Autodesk Inventor part; units mm, degrees
(part 3 of 3)
sketch "Sketch57" plane through (0, 10, 0) normal (0, 1, 0) x (1, 0, 0)
  line L0 (-74.5, 125.8) -> (-66.5, 125.8) projected
  line L1 (-83.25, 131.7) -> (2.25, 131.7) projected
  line L2 (-74.5, 125.8) -> (-66.5, 125.8)
  line L3 (-66.5, 125.8) -> (-66.5, 131.7)
  line L4 (-66.5, 131.7) -> (-74.5, 131.7)
  line L5 (-74.5, 131.7) -> (-74.5, 125.8)
  line L6 (-66.5, 9.8) -> (-74.5, 9.8) projected
  line L7 (2.25, 3.9) -> (-83.25, 3.9) projected
  line L8 (-74.5, 9.8) -> (-66.5, 9.8)
  line L9 (-66.5, 9.8) -> (-66.5, 3.9)
  line L10 (-66.5, 3.9) -> (-74.5, 3.9)
  line L11 (-74.5, 3.9) -> (-74.5, 9.8)
  line L12 (-44.5, 125.8) -> (-36.5, 125.8) projected
  line L13 (-44.5, 125.8) -> (-36.5, 125.8)
  line L14 (-36.5, 125.8) -> (-36.5, 131.7)
  line L15 (-36.5, 131.7) -> (-44.5, 131.7)
  line L16 (-44.5, 131.7) -> (-44.5, 125.8)
  line L17 (-14.5, 125.8) -> (-6.5, 125.8) projected
  line L18 (-14.5, 125.8) -> (-6.5, 125.8)
  line L19 (-6.5, 125.8) -> (-6.5, 131.7)
  line L20 (-6.5, 131.7) -> (-14.5, 131.7)
  line L21 (-14.5, 131.7) -> (-14.5, 125.8)
  line L22 (-44.5, 9.8) -> (-44.5, 125.8) projected
  line L23 (-44.5, 9.8) -> (-36.5, 9.8)
  line L24 (-36.5, 9.8) -> (-36.5, 3.9)
  line L25 (-36.5, 3.9) -> (-44.5, 3.9)
  line L26 (-44.5, 3.9) -> (-44.5, 9.8)
  line L27 (-6.5, 9.8) -> (-14.5, 9.8) projected
  line L28 (-14.5, 9.8) -> (-6.5, 9.8)
  line L29 (-6.5, 9.8) -> (-6.5, 3.9)
  line L30 (-6.5, 3.9) -> (-14.5, 3.9)
  line L31 (-14.5, 3.9) -> (-14.5, 9.8)
  point P0 (0, 0)
  dimension "d516" = 8
  dimension "d517" = 8
  constraints: 48 end point, 12 parallel, 9 point on line, 6 horizontal, 6 perpendicular
  measures "d516" distance of L4.end L3.end
  measures "d517" distance of L15.end L14.end
extrude "Extrusion53" add sketch "Sketch57" against normal blind 5
sketch "Sketch59" plane through (0, 10, 0) normal (0, 1, 0) x (1, 0, 0)
  point P0 (0, 0)
sketch "Sketch60" plane through (0, 10, 0) normal (0, 1, 0) x (1, 0, 0)
  line L0 (-66.5, 131.7) -> (-66.5, 3.9) projected
  line L1 (-66.5, 131.7) -> (-74.5, 131.7) projected
  line L2 (-74.5, 3.9) -> (-74.5, 131.7) projected
  line L3 (-74.5, 3.9) -> (-66.5, 3.9) projected
  line L4 (-36.5, 131.7) -> (-36.5, 3.9) projected
  line L5 (-36.5, 131.7) -> (-44.5, 131.7) projected
  line L6 (-44.5, 3.9) -> (-44.5, 131.7) projected
  line L7 (-44.5, 3.9) -> (-36.5, 3.9) projected
  line L8 (-6.5, 131.7) -> (-6.5, 3.9) projected
  line L9 (-6.5, 131.7) -> (-14.5, 131.7) projected
  line L10 (-14.5, 3.9) -> (-14.5, 131.7) projected
  line L11 (-14.5, 3.9) -> (-6.5, 3.9) projected
  point P0 (0, 0)
extrude "Extrusion54" add sketch "Sketch60" along normal blind 3
sketch "Sketch62" plane through (0, 13, 0) normal (0, 1, 0) x (1, 0, 0)
  line L0 (-66.5, 131.7) -> (-66.5, 3.9) projected
  line L1 (-74.5, 3.9) -> (-74.5, 131.7) projected
  line L2 (-66.5, 131.7) -> (-74.5, 131.7)
  line L3 (-74.5, 131.7) -> (-74.5, 108.7)
  line L4 (-74.5, 108.7) -> (-66.5, 108.7)
  line L5 (-66.5, 108.7) -> (-66.5, 131.7)
  line L6 (-74.5, 108.7) -> (-66.5, 108.7)
  line L7 (-66.5, 108.7) -> (-66.5, 85.7)
  line L8 (-66.5, 85.7) -> (-74.5, 85.7)
  line L9 (-74.5, 85.7) -> (-74.5, 108.7)
  line L10 (-74.5, 85.7) -> (-66.5, 85.7)
  line L11 (-66.5, 85.7) -> (-66.5, 62.7)
  line L12 (-66.5, 62.7) -> (-74.5, 62.7)
  line L13 (-74.5, 62.7) -> (-74.5, 85.7)
  line L14 (-74.5, 62.7) -> (-66.5, 62.7)
  line L15 (-66.5, 62.7) -> (-66.5, 39.7)
  line L16 (-66.5, 39.7) -> (-74.5, 39.7)
  line L17 (-74.5, 39.7) -> (-74.5, 62.7)
  line L18 (-66.5, 39.7) -> (-74.5, 39.7)
  line L19 (-74.5, 39.7) -> (-74.5, 16.7)
  line L20 (-74.5, 16.7) -> (-66.5, 16.7)
  line L21 (-66.5, 16.7) -> (-66.5, 39.7)
  line L22 (-83.25, 131.7) -> (2.25, 131.7) projected
  line L23 (-83.25, 131.7) -> (-76.85, 131.7)
  line L24 (-76.85, 131.7) -> (-76.85, 125.3)
  line L25 (-76.85, 125.3) -> (-83.25, 125.3)
  line L26 (-83.25, 125.3) -> (-83.25, 131.7)
  line L27 (2.25, 131.7) -> (2.25, 3.9) projected
  line L28 (2.25, 3.9) -> (-4.15, 3.9)
  line L29 (-4.15, 3.9) -> (-4.15, 10.3)
  line L30 (-4.15, 10.3) -> (2.25, 10.3)
  line L31 (2.25, 10.3) -> (2.25, 3.9)
  line L32 (2.25, 3.9) -> (-83.25, 3.9)
  line L33 (-83.25, 3.9) -> (-83.25, 131.7)
  line L34 (-83.25, 131.7) -> (2.25, 131.7)
  line L35 (2.25, 131.7) -> (2.25, 3.9)
  line L36 (-4.15, 10.3) -> (-76.85, 10.3)
  line L37 (-76.85, 10.3) -> (-76.85, 125.3)
  line L38 (-76.85, 125.3) -> (-4.15, 125.3)
  line L39 (-4.15, 125.3) -> (-4.15, 10.3)
  point P0 (0, 0)
  dimension "d558" = 23
  dimension "d559" = 23
  dimension "d560" = 23
  dimension "d561" = 23
  dimension "d562" = 23
  dimension "d563" = 6.4
  dimension "d564" = 6.4
  dimension "d565" = 6.4
  dimension "d566" = 6.4
  constraints: 72 end point, 18 parallel, 9 horizontal, 9 perpendicular, 5 point on line
  measures "d558" distance of L3.end L2.end
  measures "d559" distance of L6.end L7.end
  measures "d560" distance of L10.end L11.end
  measures "d561" distance of L14.end L15.end
  measures "d562" distance of L19.end L18.end
  measures "d563" distance of L24.end L25.end
  measures "d564" distance of L23.end L24.end
  measures "d565" distance of L29.end L30.end
  measures "d566" distance of L28.end L29.end
extrude "Extrusion55" cut sketch "Sketch62" against normal blind 8 contours L38 L1 L2 L0 | L0 L22 L27 L30 L39 L38 | L38 L24 L22 L1 | L25 L26 L22 L24 | L37 L36 L1 L32 L33 L25 | L30 L27 L28 L29 | L29 L32 L0 L36 | L0 L32 L1 L36
sketch "Sketch63" plane through (0, 13, 0) normal (0, 1, 0) x (1, 0, 0)
  line L0 (-66.5, 125.3) -> (-74.5, 125.3) projected
  line L1 (-6.5, 125.3) -> (-6.5, 10.3) projected
  line L2 (-74.5, 125.3) -> (-6.5, 125.3)
  line L3 (-6.5, 125.3) -> (-6.5, 102.3)
  line L4 (-6.5, 102.3) -> (-74.5, 102.3)
  line L5 (-74.5, 102.3) -> (-74.5, 125.3)
  line L6 (-74.5, 125.3) -> (-74.5, 10.3) projected
  line L7 (-6.5, 102.3) -> (-74.5, 102.3)
  line L8 (-74.5, 102.3) -> (-74.5, 79.3)
  line L9 (-74.5, 79.3) -> (-6.5, 79.3)
  line L10 (-6.5, 79.3) -> (-6.5, 102.3)
  line L11 (-74.5, 79.3) -> (-6.5, 79.3)
  line L12 (-6.5, 79.3) -> (-6.5, 56.3)
  line L13 (-6.5, 56.3) -> (-74.5, 56.3)
  line L14 (-74.5, 56.3) -> (-74.5, 79.3)
  line L15 (-6.5, 56.3) -> (-74.5, 56.3)
  line L16 (-74.5, 56.3) -> (-74.5, 33.3)
  line L17 (-74.5, 33.3) -> (-6.5, 33.3)
  line L18 (-6.5, 33.3) -> (-6.5, 56.3)
  line L19 (-74.5, 33.3) -> (-6.5, 33.3)
  line L20 (-6.5, 33.3) -> (-6.5, 10.3)
  line L21 (-6.5, 10.3) -> (-74.5, 10.3)
  line L22 (-74.5, 10.3) -> (-74.5, 33.3)
  line L23 (-66.5, 10.3) -> (-66.5, 125.3) projected
  line L24 (-74.5, 125.3) -> (-66.5, 125.3)
  line L25 (-66.5, 125.3) -> (-66.5, 102.3)
  line L26 (-66.5, 102.3) -> (-74.5, 102.3)
  line L27 (-74.5, 102.3) -> (-74.5, 125.3)
  line L28 (-74.5, 102.3) -> (-66.5, 102.3)
  line L29 (-66.5, 102.3) -> (-66.5, 79.3)
  line L30 (-66.5, 79.3) -> (-74.5, 79.3)
  line L31 (-74.5, 79.3) -> (-74.5, 102.3)
  line L32 (-74.5, 79.3) -> (-66.5, 79.3)
  line L33 (-66.5, 79.3) -> (-66.5, 56.3)
  line L34 (-66.5, 56.3) -> (-74.5, 56.3)
  line L35 (-74.5, 56.3) -> (-74.5, 79.3)
  line L36 (-74.5, 56.3) -> (-66.5, 56.3)
  line L37 (-66.5, 56.3) -> (-66.5, 33.3)
  line L38 (-66.5, 33.3) -> (-74.5, 33.3)
  line L39 (-74.5, 33.3) -> (-74.5, 56.3)
  line L40 (-74.5, 33.3) -> (-66.5, 33.3)
  line L41 (-66.5, 33.3) -> (-66.5, 10.3)
  line L42 (-66.5, 10.3) -> (-74.5, 10.3)
  line L43 (-74.5, 10.3) -> (-74.5, 33.3)
  line L44 (-44.5, 125.3) -> (-44.5, 10.3) projected
  line L45 (-36.5, 125.3) -> (-36.5, 10.3) projected
  line L46 (-44.5, 10.3) -> (-36.5, 10.3)
  line L47 (-36.5, 10.3) -> (-36.5, 33.3)
  line L48 (-36.5, 33.3) -> (-44.5, 33.3)
  line L49 (-44.5, 33.3) -> (-44.5, 10.3)
  line L50 (-44.5, 56.3) -> (-36.5, 56.3)
  line L51 (-36.5, 56.3) -> (-36.5, 33.3)
  line L52 (-36.5, 33.3) -> (-44.5, 33.3)
  line L53 (-44.5, 33.3) -> (-44.5, 56.3)
  line L54 (-44.5, 56.3) -> (-36.5, 56.3)
  line L55 (-36.5, 56.3) -> (-36.5, 79.3)
  line L56 (-36.5, 79.3) -> (-44.5, 79.3)
  line L57 (-44.5, 79.3) -> (-44.5, 56.3)
  line L58 (-44.5, 79.3) -> (-36.5, 79.3)
  line L59 (-36.5, 79.3) -> (-36.5, 102.3)
  line L60 (-36.5, 102.3) -> (-44.5, 102.3)
  line L61 (-44.5, 102.3) -> (-44.5, 79.3)
  line L62 (-44.5, 102.3) -> (-36.5, 102.3)
  line L63 (-36.5, 102.3) -> (-36.5, 125.3)
  line L64 (-36.5, 125.3) -> (-44.5, 125.3)
  line L65 (-44.5, 125.3) -> (-44.5, 102.3)
  line L66 (-14.5, 125.3) -> (-14.5, 10.3) projected
  line L67 (-6.5, 125.3) -> (-14.5, 125.3)
  line L68 (-14.5, 125.3) -> (-14.5, 102.3)
  line L69 (-14.5, 102.3) -> (-6.5, 102.3)
  line L70 (-6.5, 102.3) -> (-6.5, 125.3)
  line L71 (-6.5, 79.3) -> (-14.5, 79.3)
  line L72 (-14.5, 79.3) -> (-14.5, 102.3)
  line L73 (-14.5, 102.3) -> (-6.5, 102.3)
  line L74 (-6.5, 102.3) -> (-6.5, 79.3)
  line L75 (-14.5, 79.3) -> (-6.5, 79.3)
  line L76 (-6.5, 79.3) -> (-6.5, 56.3)
  line L77 (-6.5, 56.3) -> (-14.5, 56.3)
  line L78 (-14.5, 56.3) -> (-14.5, 79.3)
  line L79 (-14.5, 56.3) -> (-6.5, 56.3)
  line L80 (-6.5, 56.3) -> (-6.5, 33.3)
  line L81 (-6.5, 33.3) -> (-14.5, 33.3)
  line L82 (-14.5, 33.3) -> (-14.5, 56.3)
  line L83 (-14.5, 33.3) -> (-6.5, 33.3)
  line L84 (-6.5, 33.3) -> (-6.5, 10.3)
  line L85 (-6.5, 10.3) -> (-14.5, 10.3)
  line L86 (-14.5, 10.3) -> (-14.5, 33.3)
  line L87 (-70.5, 125.3) -> (-74.5, 121.3)
  line L88 (-70.5, 125.3) -> (-64.8431, 125.3) construction
  line L89 (-74.5, 121.3) -> (-70.5, 125.3)
  line L90 (-70.5, 125.3) -> (-66.5, 121.3)
  line L91 (-70.5, 102.3) -> (-66.5, 106.3)
  line L92 (-70.5, 102.3) -> (-74.5, 106.3)
  line L93 (-70.5, 102.3) -> (-66.5, 98.3)
  line L94 (-70.5, 102.3) -> (-74.5, 98.3)
  line L95 (-70.5, 79.3) -> (-66.5, 83.3)
  line L96 (-70.5, 79.3) -> (-74.5, 83.3)
  line L97 (-70.5, 79.3) -> (-66.5, 75.3)
  line L98 (-70.5, 79.3) -> (-74.5, 75.3)
  line L99 (-70.5, 56.3) -> (-66.5, 60.3)
  line L100 (-70.5, 56.3) -> (-74.5, 60.3)
  line L101 (-70.5, 56.3) -> (-74.5, 52.3)
  line L102 (-70.5, 56.3) -> (-66.5, 52.3)
  line L103 (-70.5, 33.3) -> (-66.5, 37.3)
  line L104 (-70.5, 33.3) -> (-74.5, 37.3)
  line L105 (-70.5, 33.3) -> (-74.5, 29.3)
  line L106 (-70.5, 33.3) -> (-66.5, 29.3)
  line L107 (-70.5, 10.3) -> (-74.5, 14.3)
  line L108 (-70.5, 10.3) -> (-66.5, 14.3)
  line L109 (-36.5, 125.3) -> (-44.5, 125.3) projected
  line L110 (-40.5, 125.3) -> (-44.5, 121.3)
  line L111 (-40.5, 125.3) -> (-36.5, 121.3)
  line L112 (-40.5, 102.3) -> (-36.5, 106.3)
  line L113 (-40.5, 102.3) -> (-44.5, 106.3)
  line L114 (-40.5, 102.3) -> (-44.5, 98.3)
  line L115 (-40.5, 102.3) -> (-36.5, 98.3)
  line L116 (-40.5, 79.3) -> (-44.5, 83.3)
  line L117 (-40.5, 79.3) -> (-36.5, 83.3)
  line L118 (-36.5, 83.3) -> (-40.5, 79.3)
  line L119 (-44.5, 75.3) -> (-40.5, 79.3)
  line L120 (-36.5, 75.3) -> (-40.5, 79.3)
  line L121 (-40.5, 56.3) -> (-36.5, 60.3)
  line L122 (-40.5, 56.3) -> (-44.5, 60.3)
  line L123 (-40.5, 56.3) -> (-44.5, 52.3)
  line L124 (-40.5, 56.3) -> (-36.5, 52.3)
  line L125 (-40.5, 33.3) -> (-36.5, 37.3)
  line L126 (-40.5, 33.3) -> (-44.5, 37.3)
  line L127 (-40.5, 33.3) -> (-44.5, 29.3)
  line L128 (-40.5, 33.3) -> (-36.5, 29.3)
  line L129 (-40.5, 10.3) -> (-36.5, 14.3)
  line L130 (-40.5, 10.3) -> (-44.5, 14.3)
  line L131 (-6.5, 125.3) -> (-14.5, 125.3) projected
  line L132 (-10.5, 125.3) -> (-14.5, 121.3)
  line L133 (-10.5, 125.3) -> (-6.5, 121.3)
  line L134 (-10.5, 102.3) -> (-6.5, 106.3)
  line L135 (-10.5, 102.3) -> (-4.8431, 102.3) construction
  line L136 (-6.5, 106.3) -> (-10.5, 102.3)
  line L137 (-14.5, 106.3) -> (-10.5, 102.3)
  line L138 (-10.5, 102.3) -> (-14.5, 98.3)
  line L139 (-10.5, 102.3) -> (-6.5, 98.3)
  line L140 (-10.5, 79.3) -> (-6.5, 83.3)
  line L141 (-10.5, 79.3) -> (-14.5, 83.3)
  line L142 (-10.5, 79.3) -> (-14.5, 75.3)
  line L143 (-10.5, 79.3) -> (-6.5, 75.3)
  line L144 (-10.5, 56.3) -> (-6.5, 60.3)
  line L145 (-10.5, 56.3) -> (-4.8431, 56.3) construction
  line L146 (-6.5, 60.3) -> (-10.5, 56.3)
  line L147 (-14.5, 60.3) -> (-10.5, 56.3)
  line L148 (-10.5, 56.3) -> (-14.5, 52.3)
  line L149 (-10.5, 56.3) -> (-6.5, 52.3)
  line L150 (-10.5, 33.3) -> (-6.5, 37.3)
  line L151 (-10.5, 33.3) -> (-14.5, 37.3)
  line L152 (-10.5, 33.3) -> (-14.5, 29.3)
  line L153 (-10.5, 33.3) -> (-6.5, 29.3)
  line L154 (-14.5, 10.3) -> (-6.5, 10.3) projected
  line L155 (-10.5, 10.3) -> (-6.5, 14.3)
  line L156 (-10.5, 10.3) -> (-14.5, 14.3)
  point P0 (0, 0)
  dimension "d569" = 23
  dimension "d570" = 23
  dimension "d571" = 23
  dimension "d572" = 23
  dimension "d573" = 23
  dimension "d574" = 135
  dimension "d575" = 45
  dimension "d576" = 45
  constraints: 294 end point, 109 point on line, 53 equal length, 48 perpendicular, 23 horizontal, 18 midpoint
  measures "d569" distance of L2.end L3.end
  measures "d570" distance of L8.end L7.end
  measures "d571" distance of L11.end L12.end
  measures "d572" distance of L16.end L15.end
  measures "d573" distance of L19.end L20.end
  measures "d574" angle of L87 L88
  measures "d575" angle of L135 L134
  measures "d576" angle of L145 L144
extrude "Extrusion56" cut sketch "Sketch63" against normal blind 3 contours L90 L23 L91 L92 L5 L87 | L111 L45 L112 L113 L44 L110 | L93 L23 L95 L96 L6 L94 | L115 L45 L117 L116 L44 L114 | L133 L1 L134 L137 L66 L132 | L97 L23 L99 L100 L6 L98 | L139 L1 L140 L141 L66 L138 | L120 L45 L121 L122 L44 L119 | L143 L1 L144 L147 L66 L142 | L102 L23 L103 L104 L6 L101 | L124 L45 L125 L126 L44 L123 | L149 L1 L150 L151 L66 L148 | L106 L23 L108 L107 L6 L105 | L128 L45 L129 L130 L44 L127 | L153 L1 L155 L156 L66 L152
sketch "Sketch64" plane through (0, 13, 0) normal (0, 1, 0) x (1, 0, 0)
  line L0 (-83.25, 131.7) -> (2.25, 131.7) projected
  line L1 (2.25, 131.7) -> (2.25, 3.9) projected
  line L2 (-83.25, 131.7) -> (2.25, 131.7)
  line L3 (2.25, 131.7) -> (2.25, 3.9)
  line L4 (2.25, 3.9) -> (-83.25, 3.9)
  line L5 (-83.25, 3.9) -> (-83.25, 131.7)
  point P0 (0, 0)
  constraints: 8 end point, 2 parallel, 1 horizontal, 1 perpendicular
extrude "Extrusion57" cut sketch "Sketch64" against normal blind 10
sketch "Sketch65" plane through (0, 3, 0) normal (0, 1, 0) x (1, 0, 0)
  line L0 (2.25, 3.9) -> (-83.25, 3.9) projected
  line L1 (2.25, 131.7) -> (2.25, 3.9) projected
  line L2 (-83.25, 131.7) -> (2.25, 131.7) projected
  line L3 (-83.25, 3.9) -> (-83.25, 131.7) projected
  point P0 (0, 0)
extrude "Extrusion58" add sketch "Sketch65" along normal blind 5
sketch "Sketch66" plane through (0, 8, 0) normal (0, 1, 0) x (1, 0, 0)
  point P0 (0, 0)
sketch "Sketch67" plane through (0, 8, 0) normal (0, 1, 0) x (1, 0, 0)
  point P0 (0, 0)
sketch "Sketch68" plane through (0, 8, 0) normal (0, 1, 0) x (1, 0, 0)
  line L0 (-83.25, 3.9) -> (-83.25, 131.7) projected
  line L1 (-83.25, 131.7) -> (2.25, 131.7) projected
  line L2 (-83.25, 3.9) -> (2.25, 3.9)
  line L3 (2.25, 3.9) -> (2.25, 131.7)
  line L4 (2.25, 131.7) -> (-83.25, 131.7)
  line L5 (-83.25, 131.7) -> (-83.25, 3.9)
  line L6 (2.25, 3.9) -> (-83.25, 3.9) projected
  line L7 (-40.5, 3.9) -> (-83.25, 3.9)
  line L8 (-83.25, 3.9) -> (-83.25, 131.7)
  line L9 (-83.25, 131.7) -> (-40.5, 131.7)
  line L10 (-40.5, 131.7) -> (-40.5, 3.9)
  line L11 (-83.25, 3.9) -> (-61.875, 3.9)
  line L12 (-61.875, 3.9) -> (-61.875, 131.7)
  line L13 (-61.875, 131.7) -> (-83.25, 131.7)
  line L14 (-83.25, 131.7) -> (-83.25, 3.9)
  line L15 (-61.875, 3.9) -> (-63.145, 3.9)
  line L16 (-63.145, 3.9) -> (-63.145, 131.7)
  line L17 (-63.145, 131.7) -> (-61.875, 131.7)
  line L18 (-61.875, 131.7) -> (-61.875, 3.9)
  line L19 (-63.145, 131.7) -> (-60.605, 131.7)
  line L20 (-60.605, 131.7) -> (-60.605, 3.9)
  line L21 (-60.605, 3.9) -> (-63.145, 3.9)
  line L22 (-63.145, 3.9) -> (-63.145, 131.7)
  line L23 (-63.145, 67.8) -> (-60.605, 67.8)
  line L24 (-60.605, 67.8) -> (-60.605, 86.85)
  line L25 (-60.605, 86.85) -> (-63.145, 86.85)
  line L26 (-63.145, 86.85) -> (-63.145, 67.8)
  line L27 (-60.605, 86.85) -> (-63.145, 86.85)
  line L28 (-63.145, 86.85) -> (-63.145, 48.75)
  line L29 (-63.145, 48.75) -> (-60.605, 48.75)
  line L30 (-60.605, 48.75) -> (-60.605, 86.85)
  point P0 (0, 0)
  dimension "d583" = 1.27
  dimension "d584" = 2.54
  dimension "d585" = 19.05
  dimension "d586" = 2.54
  dimension "d587" = 38.1
  constraints: 56 end point, 14 parallel, 7 horizontal, 7 perpendicular, 3 midpoint, 3 point on line
  measures "d583" distance of L16.end L17.end
  measures "d584" distance of L20.end L21.end
  measures "d585" distance of L24.end L23.end
  measures "d586" distance of L29.end L28.end
  measures "d587" distance of L28.end L27.end
extrude "Extrusion59" add sketch "Sketch68" along normal blind 50.8 contours L16 L23 L12 L29 | L25 L12 L23 L16 | L12 L23 L20 L29 | L25 L20 L23 L12
sketch "Sketch69" plane through (-63.145, 8, -86.85) normal (-1, 0, 0) x (0, 0, 1)
  line L0 (0, 50.8) -> (4.9276, 50.8)
  line L1 (4.9276, 50.8) -> (4.9276, 45.8724)
  line L2 (4.9276, 45.8724) -> (0, 45.8724)
  line L3 (0, 45.8724) -> (0, 50.8)
  line L4 (0, 50.8) -> (38.1, 50.8) projected
  line L5 (38.1, 50.8) -> (0, 50.8)
  line L6 (0, 50.8) -> (0, 12.7)
  line L7 (0, 12.7) -> (38.1, 12.7)
  line L8 (38.1, 12.7) -> (38.1, 50.8)
  line L9 (0, 12.7) -> (4.9276, 12.7)
  line L10 (4.9276, 12.7) -> (4.9276, 17.6276)
  line L11 (4.9276, 17.6276) -> (0, 17.6276)
  line L12 (0, 17.6276) -> (0, 12.7)
  line L13 (38.1, 12.7) -> (33.1724, 12.7)
  line L14 (33.1724, 12.7) -> (33.1724, 17.6276)
  line L15 (33.1724, 17.6276) -> (38.1, 17.6276)
  line L16 (38.1, 17.6276) -> (38.1, 12.7)
  line L17 (38.1, 0) -> (38.1, 50.8) projected
  line L18 (38.1, 50.8) -> (33.1724, 50.8)
  line L19 (33.1724, 50.8) -> (33.1724, 45.8724)
  line L20 (33.1724, 45.8724) -> (38.1, 45.8724)
  line L21 (38.1, 45.8724) -> (38.1, 50.8)
  line L22 (38.1, 50.8) -> (19.05, 50.8)
  line L23 (19.05, 50.8) -> (19.05, 31.75)
  line L24 (19.05, 31.75) -> (38.1, 31.75)
  line L25 (38.1, 31.75) -> (38.1, 50.8)
  circle A0 centre (19.05, 31.75) radius 11.43
  circle A1 centre (33.1724, 45.8724) radius 1.27
  circle A2 centre (4.9276, 45.8724) radius 1.27
  circle A3 centre (4.9276, 17.6276) radius 1.27
  circle A4 centre (33.1724, 17.6276) radius 1.27
  point P0 (86.85, -8)
  dimension "d590" = 4.9276
  dimension "d591" = 4.9276
  dimension "d592" = 38.1
  dimension "d593" = 38.1
  dimension "d594" = 4.9276
  dimension "d595" = 4.9276
  dimension "d596" = 4.9276
  dimension "d597" = 4.9276
  dimension "d598" = 4.9276
  dimension "d599" = 4.9276
  dimension "d600" = 19.05
  dimension "d601" = 19.05
  dimension "d602" = 22.86
  dimension "d603" = 2.54
  dimension "d604" = 2.54
  dimension "d605" = 2.54
  dimension "d606" = 2.54
  constraints: 48 end point, 12 parallel, 6 horizontal, 6 perpendicular, 5 centre point, 5 coincident
  measures "d590" distance of L1.end L2.end
  measures "d591" distance of L0.end L1.end
  measures "d592" distance of L7.end L6.end
  measures "d593" distance of L6.end L5.end
  measures "d594" distance of L11.end L10.end
  measures "d595" distance of L10.end L9.end
  measures "d596" distance of L14.end L15.end
  measures "d597" distance of L13.end L14.end
  measures "d598" distance of L20.end L19.end
  measures "d599" distance of L19.end L18.end
  measures "d600" distance of L24.end L23.end
  measures "d601" distance of L23.end L22.end
  measures "d602" diameter of A0
  measures "d603" diameter of A1
  measures "d604" diameter of A2
  measures "d605" diameter of A3
  measures "d606" diameter of A4
extrude "Extrusion60" cut sketch "Sketch69" against normal blind 50.8 contours A2 L2 L1 | L1 L2 A2 | A0 L24 L23 | L23 L24 A0 | A3 L10 L11 | L11 L10 A3 | A1 L20 L19 | L19 L20 A1 | A4 L15 L14 | L14 L15 A4
sketch "Sketch70" plane through (0, 8, 0) normal (0, 1, 0) x (1, 0, 0)
  line L0 (2.25, 3.9) -> (2.25, 131.7) projected
  line L1 (2.25, 131.7) -> (-83.25, 131.7) projected
  line L2 (2.25, 3.9) -> (-2.83, 3.9)
  line L3 (-2.83, 3.9) -> (-2.83, 131.7)
  line L4 (-2.83, 131.7) -> (2.25, 131.7)
  line L5 (2.25, 131.7) -> (2.25, 3.9)
  point P0 (0, 0)
  dimension "d609" = 5.08
  constraints: 8 end point, 2 parallel, 1 horizontal, 1 perpendicular, 1 point on line
  measures "d609" distance of L3.end L4.end
extrude "Extrusion61" add sketch "Sketch70" along normal blind 76.2
body "Solid1"
